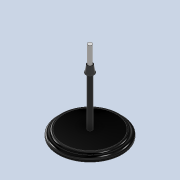
# Autodesk Inventor part: Base
Saved by Autodesk Inventor 2021 (Build 250183000, 183)
## iProperties
Created: 2020-07-20
Part Number: Base
Material: Generic
Document SubType Name: Modeling
Designer: brook
Density: 1 g/cm^3
Appearance: Default
Author: brook
Autodesk Inventor part; units mm, degrees
ref_plane "YZ Plane" through (0, 0, 0) normal (1, 0, 0) x (0, 1, 0)
ref_plane "XZ Plane" through (0, 0, 0) normal (0, 1, 0) x (-1, 0, 0)
ref_plane "XY Plane" through (0, 0, 0) normal (0, 0, 1) x (1, 0, 0)
sketch "Sketch1" plane through (0, 0, 0) normal (1, 0, 0) x (0, 1, 0)
  line L0 (0, 0) -> (0, 235)
  line L1 (0, 235) -> (15, 235)
  arc A0 (15, 235) -> (31.9412, 215.2353) centre (35, 235) ccw
  arc A1 (45, 200) -> (31.9412, 215.2353) centre (29.5833, 200) ccw
  line L2 (45, 200) -> (45, 195)
  line L3 (45, 195) -> (44, 195)
  line L4 (44, 195) -> (44, 193)
  line L5 (44, 193) -> (45, 193)
  line L6 (45, 193) -> (45, 0)
  line L7 (45, 0) -> (0, 0)
  dimension "d0" = 235
  dimension "d1" = 195
  dimension "d2" = 15
  dimension "d3" = 2
  dimension "d4" = 1
  dimension "d5" = 30
  dimension "d6" = 200
  dimension "d7" = 20
  constraints: 16 end point, 5 perpendicular, 4 point on circle, 2 centre point, 2 point on line, 2 tangent, 2 vertical, 1 line through centre
  measures "d0" distance of L0.start L0.end
  measures "d1" distance between parallel lines of L3 L7
  measures "d2" distance of L0.end L1.end
  measures "d3" distance between parallel lines of L5 L3
  measures "d4" distance of L4.end L5.end
  measures "d5" distance from line of L2 L1.end
  measures "d6" distance from line of L7 L2.start
  measures "d7" radius of A0
revolve "Revolution1" add sketch "Sketch1" angle 360 about axis through (0, 45, 0) along (0, -1, 0)
sketch "Sketch2" plane through (0, 45, 0) normal (0, 1, 0) x (1, 0, 0)
  circle A0 centre (0, 0) radius 17.5
  dimension "d9" = 35
  constraints: 1 centre point, 1 coincident
  measures "d9" diameter of A0
extrude "Extrusion1" add sketch "Sketch2" along normal blind 415
sketch "Sketch3" plane through (0, 0, 0) normal (1, 0, 0) x (0, 1, 0)
  line L0 (405, -25) -> (405, -30)
  line L1 (405, -30) -> (410, -30)
  line L2 (410, -30) -> (410, -28)
  line L3 (410, -28) -> (460, -20.5)
  line L4 (460, -20.5) -> (460, 0)
  line L5 (460, 0) -> (455, 0)
  line L6 (455, 0) -> (455, -17.5)
  line L7 (455, -17.5) -> (405, -25)
  line L8 (45, 17.5) -> (45, -17.5) projected
  line L9 (-119, 0) -> (714, 0) projected
  point P0 (0, 0)
  dimension "d12" = 5
  dimension "d13" = 360
  dimension "d14" = 5
  dimension "d15" = 50
  dimension "d16" = 2
  dimension "d17" = 55
  dimension "d18" = 0
  dimension "d19" = 30
  dimension "d20" = 17.5
  constraints: 16 end point, 4 perpendicular, 2 vertical, 1 parallel
  measures "d12" distance of L0.start L0.end
  measures "d13" distance between parallel lines of L8 L0
  measures "d14" distance of L0.end L1.end
  measures "d15" distance between parallel lines of L0 L6
  measures "d16" distance of L1.end L2.end
  measures "d17" distance between parallel lines of L0 L4
  measures "d18" distance from line of point (0, 0) L5
  measures "d19" distance between parallel lines of L5 L1
  measures "d20" distance from line of L5 L6.end
revolve "Revolution2" add sketch "Sketch3" angle 360 about axis through (0, -10, 0) along (0, 1, 0)
sketch "Sketch6" plane through (0, 460, 0) normal (0, 1, 0) x (1, 0, 0)
  circle A0 centre (0, 0) radius 15
  dimension "d27" = 30
  constraints: 1 centre point, 1 coincident
  measures "d27" diameter of A0
extrude "Extrusion3" add sketch "Sketch6" along normal blind 130
body "Solid1"
